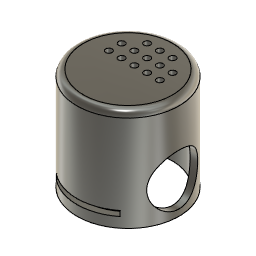
CoopForHamsters (Autodesk Fusion 360 design; units mm, degrees)
Autodesk Fusion 360 part; units mm, degrees
sketch "スケッチ1" plane through (0, 0, 0) normal (0, 0, 1) x (1, 0, 0)
  circle A0 centre (0, 0) radius 40
  constraint coincident A0.centre origin
extrude "押し出し1" add sketch "スケッチ1" along normal blind 80
shell "シェル1" thickness 5 removed faces 1 at (9.4847, -14.2223, 0)
fillet "フィレット1" radius 5 1 edges at (-37.2931, -14.4646, 80)
ref_plane "作業平面1" through (45, 0, 0) normal (1, 0, 0) x (0, 1, 0)
sketch "スケッチ2" plane through (45, 0, 0) normal (1, 0, 0) x (0, 1, 0)
  circle A0 centre (0, 25) radius 20
extrude "押し出し2" cut sketch "スケッチ2" against normal blind 25
sketch "スケッチ3" plane through (0, 0, 80) normal (0, 0, 1) x (-1, 0, 0)
  circle A0 centre (0, 0) radius 35
  circle A1 centre (10, -25) radius 2.5
  circle A2 centre (0, -25) radius 2.5
  circle A3 centre (-10, -25) radius 2.5
  circle A4 centre (10, -15) radius 2.5
  circle A5 centre (0, -15) radius 2.5
  circle A6 centre (-10, -15) radius 2.5
  circle A7 centre (-20, -15) radius 2.5
  circle A8 centre (20, -15) radius 2.5
  circle A9 centre (0, -5) radius 2.5
  circle A10 centre (-10, -5) radius 2.5
  circle A11 centre (-20, -5) radius 2.5
  circle A12 centre (10, -5) radius 2.5
  circle A13 centre (20, -5) radius 2.5
  dimension "d9" = 5
  dimension "d10" = 5
  dimension "d11" = 5
  dimension "d12" = 5
  dimension "d13" = 5
  dimension "d14" = 5
  dimension "d15" = 5
  dimension "d16" = 5
  dimension "d17" = 5
  dimension "d18" = 5
  dimension "d19" = 5
  dimension "d20" = 5
  dimension "d21" = 5
  measures "d9" diameter of A1
  measures "d10" diameter of A2
  measures "d11" diameter of A3
  measures "d12" diameter of A4
  measures "d13" diameter of A5
  measures "d14" diameter of A6
  measures "d15" diameter of A7
  measures "d16" diameter of A8
  measures "d17" diameter of A9
  measures "d18" diameter of A10
  measures "d19" diameter of A11
  measures "d20" diameter of A12
  measures "d21" diameter of A13
extrude "押し出し3" cut sketch "スケッチ3" against normal blind 8 contours A1 | A2 | A3 | A4 | A5 | A6 | A7 | A8 | A9 | A10 | A11 | A12 | A13
ref_plane "作業平面2" through (0, -45, 0) normal (0, 1, 0) x (0, 0, 1)
sketch "スケッチ4" plane through (0, -45, 0) normal (0, 1, 0) x (1, 0, 0)
  line L0 (-25, -12.0407) -> (25, -12.0407)
  line L1 (25, -12.0407) -> (25, -7.9593)
  line L2 (25, -7.9593) -> (-25, -7.9593)
  line L3 (-25, -7.9593) -> (-25, -12.0407)
  line L4 (-25, -12.0407) -> (25, -7.9593) construction
  line L5 (25, -12.0407) -> (-25, -7.9593) construction
  point P0 (0, -10)
  dimension "d25" = 50
  constraint horizontal L0
  constraint perpendicular L0 L1
  constraint parallel L0 L2
  constraint parallel L1 L3
  constraint coincident L4 P0
  constraint coincident L5 P0
  measures "d25" distance of L1.end L2.end
extrude "押し出し4" cut sketch "スケッチ4" along normal blind 30
